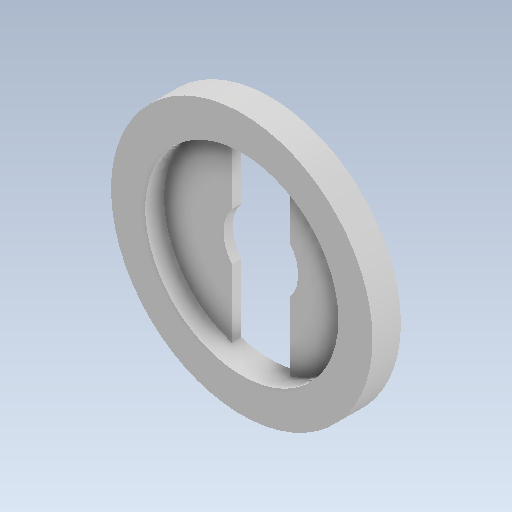
# Autodesk Inventor part: Деталь2
Saved by Autodesk Inventor 2020 (Build 240168000, 168)
## iProperties
Created: 2023-05-30
Part Number: Деталь2
Material: Типовые
Document SubType Name: Modeling
Designer: Qwellert
Density: 1 g/cm^3
Appearance: По умолчанию
Author: Qwellert
Autodesk Inventor part; units mm, degrees
ref_plane "YZ Plane" through (0, 0, 0) normal (1, 0, 0) x (0, 1, 0)
ref_plane "XZ Plane" through (0, 0, 0) normal (0, 1, 0) x (-1, 0, 0)
ref_plane "XY Plane" through (0, 0, 0) normal (0, 0, 1) x (1, 0, 0)
sketch "Эскиз1" plane through (0, 0, 0) normal (0, 0, 1) x (1, 0, 0)
  circle A0 centre (0, 0) radius 13.8038
  circle A1 centre (0, 0) radius 9.815 projected
  line L0 (-3.05, 2.51) -> (-3.05, 9.3291) projected
  line L1 (3.05, 9.3291) -> (3.05, 2.51) projected
  line L2 (-3.05, -9.3291) -> (-3.05, -2.51) projected
  line L3 (3.05, -2.51) -> (3.05, -9.3291) projected
  line L4 (-3.05, -2.51) -> (-3.05, 2.51)
  line L5 (3.05, -2.51) -> (3.05, 2.51)
  circle A2 centre (0, 0) radius 10.1941
  constraints: 4 end point, 2 centre point, 2 coincident, 1 collinear, 1 parallel
extrude "Выдавливание1" add sketch "Эскиз1" along normal blind 3 contours A0
sketch "Эскиз2" plane through (0, 0, 0) normal (0, 0, -1) x (-1, 0, 0)
  line L0 (-3.05, 9.3291) -> (-3.05, 2.51) projected
  circle A0 centre (0, 0) radius 3.95 projected
  line L1 (-3.05, -2.51) -> (-3.05, -9.3291) projected
  line L2 (3.05, -9.3291) -> (3.05, -2.51) projected
  line L3 (3.05, 2.51) -> (3.05, 9.3291) projected
  line L4 (-3.05, -9.3291) -> (-3.05, -9.7271)
  circle A1 centre (0, 0) radius 10.1941 projected
  line L5 (3.05, -9.3291) -> (3.05, -9.7271)
  line L6 (-3.05, 9.3291) -> (-3.05, 9.7271)
  line L7 (3.05, 9.3291) -> (3.05, 9.7271)
  constraints: 8 end point, 4 point on circle, 2 point on line, 1 parallel, 1 vertical
extrude "Выдавливание2" add sketch "Эскиз2" against normal blind 1 contours L0 A0 L1 L4 A1 L6 | L3 L7 A1 L5 L2 A0
